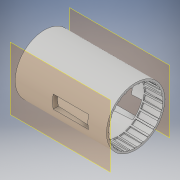
# Autodesk Inventor part: venturivalveajuster
Saved by Autodesk Inventor 2019.1 (Build 231200000, 200)
## iProperties
Created: 2020-03-22
Part Number: venturivalveajuster
Material: Generic
Document SubType Name: Modeling
Designer: Computus
Density: 1 g/cm^3
Appearance: Default
Author: Computus
## iProperties of the stored document venturivalveajuster_3DPrint.ipt
Created: 2020-03-22
Part Number: venturivalveajuster_3DPrint
Material: Generic
Document SubType Name: Modeling
Designer: Computus
Density: 1 g/cm^3
Appearance: Default
Author: Computus
Autodesk Inventor part; units mm, degrees
ref_plane "YZ Plane" through (0, 0, 0) normal (1, 0, 0) x (0, 1, 0)
ref_plane "XZ Plane" through (0, 0, 0) normal (0, 1, 0) x (-1, 0, 0)
sketch "Sketch1" plane through (0, 0, 0) normal (0, 1, 0) x (-1, 0, 0)
  line L0 (0, 10.75) -> (36.8, 9)
  line L1 (0, 10.75) -> (0, 11.75)
  line L2 (0, 11.75) -> (36.8, 11.75)
  line L3 (36.8, 11.75) -> (36.8, 9)
  line L4 (44.16, 0) -> (-7.36, 0) projected
  point P0 (0, 0)
  dimension "d29" = 9
  constraints: 8 end point, 2 perpendicular
  measures "d29" distance from line of L0.end L4
revolve "Revolution1" add sketch "Sketch1" angle 360 about axis through (-10, 0, 0) along (1, 0, 0)
sketch "Sketch2" plane through (0, 0, 0) normal (1, 0, 0) x (0, 0, -1)
  line L0 (-1, 10.1231) -> (1, 10.1231)
  line L1 (1, 10.1231) -> (1, 10.9669)
  line L2 (1, 10.9669) -> (-1, 10.9669)
  line L3 (-1, 10.9669) -> (-1, 10.1231)
  line L4 (0, -16.45) -> (0, 16.45) projected
  line L5 (-3.4861, 9.5564) -> (-1.5489, 10.0537)
  line L6 (-1.5489, 10.0537) -> (-1.7588, 10.871)
  line L7 (-1.7588, 10.871) -> (-3.6959, 10.3736)
  line L8 (-3.6959, 10.3736) -> (-3.4861, 9.5564)
  line L9 (-5.7531, 8.3892) -> (-4.0005, 9.3527)
  line L10 (-4.0005, 9.3527) -> (-4.407, 10.0921)
  line L11 (-4.407, 10.0921) -> (-6.1596, 9.1286)
  line L12 (-6.1596, 9.1286) -> (-5.7531, 8.3892)
  line L13 (-7.6587, 6.6949) -> (-6.2008, 8.064)
  line L14 (-6.2008, 8.064) -> (-6.7784, 8.679)
  line L15 (-6.7784, 8.679) -> (-8.2363, 7.3099)
  line L16 (-8.2363, 7.3099) -> (-7.6587, 6.6949)
  line L17 (-9.083, 4.5799) -> (-8.0114, 6.2686)
  line L18 (-8.0114, 6.2686) -> (-8.7238, 6.7207)
  line L19 (-8.7238, 6.7207) -> (-9.7954, 5.032)
  line L20 (-9.7954, 5.032) -> (-9.083, 4.5799)
  line L21 (-9.9366, 2.1772) -> (-9.3186, 4.0793)
  line L22 (-9.3186, 4.0793) -> (-10.1211, 4.34)
  line L23 (-10.1211, 4.34) -> (-10.7391, 2.4379)
  line L24 (-10.7391, 2.4379) -> (-9.9366, 2.1772)
  line L25 (-10.1659, -0.3624) -> (-10.0403, 1.6337)
  line L26 (-10.0403, 1.6337) -> (-10.8824, 1.6866)
  line L27 (-10.8824, 1.6866) -> (-11.008, -0.3094)
  line L28 (-11.008, -0.3094) -> (-10.1659, -0.3624)
  line L29 (-9.7564, -2.8792) -> (-10.1312, -0.9146)
  line L30 (-10.1312, -0.9146) -> (-10.96, -1.0727)
  line L31 (-10.96, -1.0727) -> (-10.5852, -3.0373)
  line L32 (-10.5852, -3.0373) -> (-9.7564, -2.8792)
  line L33 (-8.7339, -5.215) -> (-9.5854, -3.4054)
  line L34 (-9.5854, -3.4054) -> (-10.3489, -3.7646)
  line L35 (-10.3489, -3.7646) -> (-9.4973, -5.5743)
  line L36 (-9.4973, -5.5743) -> (-8.7339, -5.215)
  line L37 (-7.1626, -7.2232) -> (-8.4374, -5.6822)
  line L38 (-8.4374, -5.6822) -> (-9.0875, -6.22)
  line L39 (-9.0875, -6.22) -> (-7.8127, -7.7611)
  line L40 (-7.8127, -7.7611) -> (-7.1626, -7.2232)
  line L41 (-5.1412, -8.7775) -> (-6.7592, -7.602)
  line L42 (-6.7592, -7.602) -> (-7.2552, -8.2846)
  line L43 (-7.2552, -8.2846) -> (-5.6371, -9.4602)
  line L44 (-5.6371, -9.4602) -> (-5.1412, -8.7775)
  line L45 (-2.7968, -9.7803) -> (-4.6563, -9.0441)
  line L46 (-4.6563, -9.0441) -> (-4.9669, -9.8286)
  line L47 (-4.9669, -9.8286) -> (-3.1074, -10.5648)
  line L48 (-3.1074, -10.5648) -> (-2.7968, -9.7803)
  line L49 (-0.2766, -10.1686) -> (-2.2609, -9.9179)
  line L50 (-2.2609, -9.9179) -> (-2.3666, -10.755)
  line L51 (-2.3666, -10.755) -> (-0.3824, -11.0057)
  line L52 (-0.3824, -11.0057) -> (-0.2766, -10.1686)
  line L53 (2.2609, -9.9179) -> (0.2766, -10.1686)
  line L54 (0.2766, -10.1686) -> (0.3824, -11.0057)
  line L55 (0.3824, -11.0057) -> (2.3666, -10.755)
  line L56 (2.3666, -10.755) -> (2.2609, -9.9179)
  line L57 (4.6563, -9.0441) -> (2.7968, -9.7803)
  line L58 (2.7968, -9.7803) -> (3.1074, -10.5648)
  line L59 (3.1074, -10.5648) -> (4.9669, -9.8286)
  line L60 (4.9669, -9.8286) -> (4.6563, -9.0441)
  line L61 (6.7592, -7.602) -> (5.1412, -8.7775)
  line L62 (5.1412, -8.7775) -> (5.6371, -9.4602)
  line L63 (5.6371, -9.4602) -> (7.2552, -8.2846)
  line L64 (7.2552, -8.2846) -> (6.7592, -7.602)
  line L65 (8.4374, -5.6822) -> (7.1626, -7.2232)
  line L66 (7.1626, -7.2232) -> (7.8127, -7.7611)
  line L67 (7.8127, -7.7611) -> (9.0875, -6.22)
  line L68 (9.0875, -6.22) -> (8.4374, -5.6822)
  line L69 (9.5854, -3.4054) -> (8.7339, -5.215)
  line L70 (8.7339, -5.215) -> (9.4973, -5.5743)
  line L71 (9.4973, -5.5743) -> (10.3489, -3.7646)
  line L72 (10.3489, -3.7646) -> (9.5854, -3.4054)
  line L73 (10.1312, -0.9146) -> (9.7564, -2.8792)
  line L74 (9.7564, -2.8792) -> (10.5852, -3.0373)
  line L75 (10.5852, -3.0373) -> (10.96, -1.0727)
  line L76 (10.96, -1.0727) -> (10.1312, -0.9146)
  line L77 (10.0403, 1.6337) -> (10.1659, -0.3624)
  line L78 (10.1659, -0.3624) -> (11.008, -0.3094)
  line L79 (11.008, -0.3094) -> (10.8824, 1.6866)
  line L80 (10.8824, 1.6866) -> (10.0403, 1.6337)
  line L81 (9.3186, 4.0793) -> (9.9366, 2.1772)
  line L82 (9.9366, 2.1772) -> (10.7391, 2.4379)
  line L83 (10.7391, 2.4379) -> (10.1211, 4.34)
  line L84 (10.1211, 4.34) -> (9.3186, 4.0793)
  line L85 (8.0114, 6.2686) -> (9.083, 4.5799)
  line L86 (9.083, 4.5799) -> (9.7954, 5.032)
  line L87 (9.7954, 5.032) -> (8.7238, 6.7207)
  line L88 (8.7238, 6.7207) -> (8.0114, 6.2686)
  line L89 (6.2008, 8.064) -> (7.6587, 6.6949)
  line L90 (7.6587, 6.6949) -> (8.2363, 7.3099)
  line L91 (8.2363, 7.3099) -> (6.7784, 8.679)
  line L92 (6.7784, 8.679) -> (6.2008, 8.064)
  line L93 (4.0005, 9.3527) -> (5.7531, 8.3892)
  line L94 (5.7531, 8.3892) -> (6.1596, 9.1286)
  line L95 (6.1596, 9.1286) -> (4.407, 10.0921)
  line L96 (4.407, 10.0921) -> (4.0005, 9.3527)
  line L97 (1.5489, 10.0537) -> (3.4861, 9.5564)
  line L98 (3.4861, 9.5564) -> (3.6959, 10.3736)
  line L99 (3.6959, 10.3736) -> (1.7588, 10.871)
  line L100 (1.7588, 10.871) -> (1.5489, 10.0537)
  point P0 (0, 0)
  dimension "d4" = 2
  dimension "d5" = 1
  dimension "d8" = 360
  constraints: 200 end point, 2 parallel, 1 horizontal, 1 perpendicular, 201 other
  measures "d4" distance of L2.end L1.end
  measures "d5" distance between parallel lines of L1 L4
extrude "Extrusion1" cut sketch "Sketch2" against normal blind 7
ref_plane "Work Plane1" through (0, 0, 12) normal (0, 0, 1) x (1, 0, 0)
sketch "Sketch3" plane through (0, 0, 12) normal (0, 0, 1) x (1, 0, 0)
  line L0 (-7.5, -2.65) -> (-21.75, -2.65)
  line L1 (-21.75, -2.65) -> (-21.75, 2.65)
  line L2 (-21.75, 2.65) -> (-7.5, 2.65)
  line L3 (-7.5, 2.65) -> (-7.5, -2.65)
  line L4 (-26.1, 0) -> (4.35, 0) projected
  line L5 (0, 11.75) -> (0, -11.75) projected
  point P0 (0, 0)
  dimension "d13" = 14.25
  dimension "d14" = 5.3
  dimension "d15" = 2.65
  dimension "d16" = 7.5
  constraints: 8 end point, 2 parallel, 1 horizontal, 1 perpendicular
  measures "d13" distance of L1.end L2.end
  measures "d14" distance of L0.end L1.end
  measures "d15" distance between parallel lines of L2 L4
  measures "d16" distance between parallel lines of L5 L3
extrude "Extrusion2" cut sketch "Sketch3" against normal blind 10
ref_plane "Work Plane2" through (0, 0, -12) normal (0, 0, 1) x (1, 0, 0)
sketch "Sketch4" plane through (0, 0, -12) normal (0, 0, 1) x (1, 0, 0)
  line L0 (-7.5, -8.2172) -> (-31.5, -8.2172)
  line L1 (-31.5, -8.2172) -> (-31.5, -2.9672)
  line L2 (-11.5, -2.9672) -> (-7.5, -2.9672)
  line L3 (-7.5, -2.9672) -> (-7.5, -8.2172)
  line L4 (0, 11.75) -> (0, -11.75) projected
  line L5 (-11.5, -2.9672) -> (-11.5, 7.5328)
  line L6 (-11.5, 7.5328) -> (-31.5, 7.5328)
  line L7 (-31.5, 7.5328) -> (-31.5, -2.9672)
  point P0 (0, 0)
  constraints: 14 end point, 3 parallel, 1 horizontal, 1 perpendicular
extrude "Extrusion3" cut sketch "Sketch4" along normal blind 10
sketch "Sketch5" plane through (0, 0, -12) normal (0, 0, 1) x (1, 0, 0)
  line L0 (0, 0) -> (-2.8191, 1.0261)
  line L1 (0, 0) -> (3, 0) construction
  line L2 (0, 0) -> (-2.8191, -1.0261)
  line L3 (0, 0) -> (3, 0) construction
  line L4 (0, -1.0727) -> (-7, -1.0727) projected
  line L5 (-2.8191, -1.0261) -> (-2.8191, 1.0261)
  point P0 (-7, 1.6491)
  dimension "d30" = 3
  dimension "d31" = 160
  dimension "d32" = 3
  dimension "d33" = 160
  constraints: 10 end point, 2 equal length, 2 horizontal
  measures "d30" distance of L0.start L0.end
  measures "d31" angle of L1 L0
  measures "d32" distance of L0.start L2.end
  measures "d33" angle of L2 L3
extrude "Extrusion4" add sketch "Sketch5" along normal blind 1
body "Solid1"
